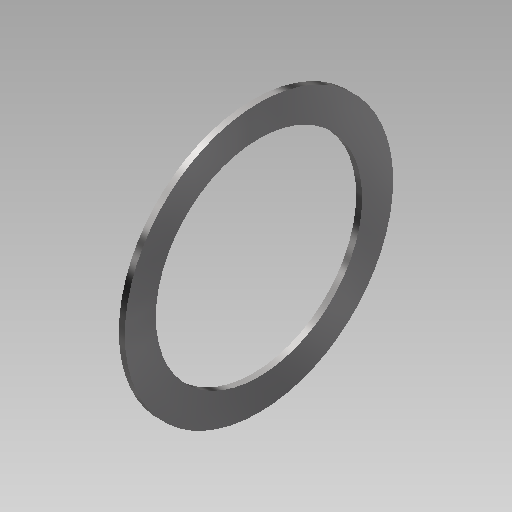
# Autodesk Inventor part: LF-1060ZZ_shield
Saved by Autodesk Inventor 2021 (Build 250183000, 183)
## iProperties
Created: 2019-09-04
Part Number: LF-1060ZZ_shield
Material: 鋼、炭素鋼
Catalog Web Link: www.cadenas.de
Description: Radial Flanged Ball Bearings (RF-Series/LF series) Metric ST shield-Radial Flanged Ball Bearings (RF-Series/LF series) Metric Shielded Type
Vendor: NMB
Document SubType Name: Modeling
Designer: psadmin
Manufacturer: NMB
Mass: 0.0412083 g
Surface Area: 0.625414 cm^2
Volume: 0.00524946 cm^3
Density: 7.85 g/cm^3
Appearance: 半つや出し
Category: PARTsolutions
Company: NMB
PSOL_IDENT_0: {$CADENAS_DATA\23d-libs\nmb\pbbp\radial_flanged_ball_bearings\rfbb_rflfs_m\rflf_shielded_shield.prj}
PSOL_IDENT_1: ,235 {VTYP=3D},{NB=LF-1060ZZ_shield},{LINA=LF-1060ZZ_shield},{NN=Radial Flanged Ball Bearings (RF-Se
PSOL_IDENT_2: ries/LF series) Metric ST shield},{DATE=11.11.2013 05:13:45},{GEOMDATE=24.10.2013 09:56:00},{VERSION=
PSOL_IDENT_3: },{LINEID=1200},{WBVAR=},{WBNUMERIC=}  {NB=LF-1060ZZ_shield},{LINA=LF-1060ZZ_shield},{KT=DUMMY},{IDN
PSOL_IDENT_4: R=},{PN=LF-1060ZZ},{SHLD=shielded},{FLANG=flanged},{SD=6.000},{D=10.000},{B=3.000},{SR=0.10},{BCZ=9}
PSOL_IDENT_5: ,{DW=1.1906},{LI=6.95},{LO=9.04},{D1=11.200},{C1=0.60},{D2=0.0},{C2=0.00},{COR=194},{CR=1029},{PCD=8
PSOL_IDENT_6: .000},{U=9.191},{W=6.809},{Y=0.595},{Z=0.595},{AA=9.072},{AC=0.60},{AD=0.000},{AF=0.00},{AQ=0.20},{A
PSOL_IDENT_7: H=9.24},{AI=7.15},{AJ=0.40}
NN: Radial Flanged Ball Bearings (RF-Series/LF series) Metric ST shield
NT: Radial Flanged Ball Bearings (RF-Series/LF series) Metric Shielded Type
NB: LF-1060ZZ_shield
NBSYN: $PN._shield
LINA: LF-1060ZZ_shield
PN: LF-1060ZZ
SHLD: shielded
FLANG: flanged
SD: 6
D: 10
B: 3
SR: 0.1
BCZ: 9
DW: 1.1906
LI: 6.95
LO: 9.04
D1: 0
C1: 0.6
D2: 0
C2: 0
COR: 194
CR: 1029
PCD: 8
U: 9.191
W: 6.809
Y: 0.595
Z: 0.595
AA: 9.072
AC: 0.6
AD: 0
AF: 0
AQ: 0.2
AH: 9.24
AI: 7.15
AJ: 0.4
SUPPLIER: NMB
ARTICLENO: LF-1060ZZ_shield
BOMINFO: LF-1060ZZ_shield
CREATOR: CADENAS GmbH
Title: LF-1060ZZ_shield
Author: Cadenas PARTsolutions
Comments: Radial Flanged Ball Bearings (RF-Series/LF series) Metric Shielded Type
Autodesk Inventor part; units mm, degrees
sketch "Sketch_1" plane through (0, 0, 0) normal (0, 0, 1) x (1, 0, 0)
  line L0 (0.2, 0) -> (0, 0)
  line L1 (0, 4.52) -> (0, 3.475)
  line L2 (0, 3.475) -> (0.2, 3.475)
  line L3 (0.2, 3.475) -> (0.2, 4.52)
  line L4 (0.2, 4.52) -> (0, 4.52)
  constraints: 10 end point
revolve "Revolution1" add sketch "Sketch_1" angle 360 about axis through (0.2, 0, 0) along (1, 0, 0)
ref_plane "1_XY" through (0, 0, 0) normal (1, 0, 0) x (0, 0, -1)
ref_plane "1_YZ" through (0, 0, 0) normal (0, 0, -1) x (0, 1, 0)
ref_plane "1_ZX" through (0, 0, 0) normal (0, 1, 0) x (1, 0, 0)
body "Solid1"
